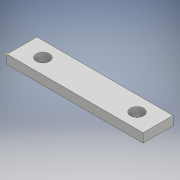
# Autodesk Inventor part: pipeServo
Saved by Autodesk Inventor 2017 (Build 210142000, 142)
## iProperties
Created: 2017-04-18
Part Number: pipeServo
Material: Generic
Document SubType Name: Modeling
Designer: s4461999
Density: 1 g/cm^3
Appearance: Default
Author: s4461999
Autodesk Inventor part; units mm, degrees
ref_plane "YZ Plane" through (0, 0, 0) normal (1, 0, 0) x (0, 1, 0)
ref_plane "XZ Plane" through (0, 0, 0) normal (0, 1, 0) x (-1, 0, 0)
ref_plane "XY Plane" through (0, 0, 0) normal (0, 0, 1) x (1, 0, 0)
sketch "Sketch1" plane through (0, 0, 0) normal (0, 0, 1) x (1, 0, 0)
  line L0 (0, 0) -> (45.5, 0)
  line L1 (45.5, 0) -> (45.5, 10)
  line L2 (45.5, 10) -> (0, 10)
  line L3 (0, 10) -> (0, 0)
  dimension "d0" = 45.5
  dimension "d1" = 10
  constraints: 8 end point, 3 perpendicular, 1 horizontal
  measures "d0" distance between parallel lines of L1 L3
  measures "d1" distance between parallel lines of L0 L2
extrude "Extrusion1" add sketch "Sketch1" along normal blind 3
sketch "Sketch2" plane through (0, 0, 3) normal (0, 0, 1) x (1, 0, 0)
  line L0 (0, 10) -> (0, 0) projected
  line L1 (45.5, 0) -> (45.5, 10) projected
  line L2 (45.5, 10) -> (0, 10) projected
  point P0 (7, 5)
  point P1 (38.5, 5)
  dimension "d4" = 7
  dimension "d5" = 7
  dimension "d6" = 5
  dimension "d7" = 5
  measures "d4" distance from line of L0 point (7, 5)
  measures "d5" distance from line of point (38.5, 5) L1
  measures "d6" distance from line of L2 point (7, 5)
  measures "d7" distance from line of L2 point (38.5, 5)
sketch "Sketch3" plane through (0, 0, 3) normal (0, 0, 1) x (1, 0, 0)
  point P0 (0, 0)
hole "Hole1" at (7, 5, 3) at (38.5, 5, 3) direction (0, 0, -1) diameter 4.4 end through all
body "Solid1"
